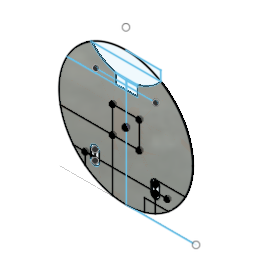
cima (Autodesk Fusion 360 archive; units mm, degrees)
design "BaseChapaCima"
Autodesk Fusion 360 part; units mm, degrees
sketch "Sketch1" plane through (0, 0, 0) normal (0, 0, -1) x (1, 0, 0)
  circle A0 centre (0, 0) radius 240
  line L0 (0.0048, -240) -> (125.0048, -240)
  line L1 (125.0048, -240) -> (125.0048, -204.8751)
  line L2 (1.5986, 239.9947) -> (1.5986, -147.0053)
  line L3 (125.0048, -204.8751) -> (-125.0048, -204.8751)
  arc A1 (125.0048, -204.8751) -> (-125.0048, -204.8751) centre (0, -310.93) ccw
  circle A2 centre (-47.294, 47.294) radius 5
  line L4 (-47.294, 47.294) -> (48.706, 47.294)
  line L5 (48.706, 47.294) -> (48.706, -48.706)
  line L6 (48.706, -48.706) -> (-47.294, -48.706)
  line L7 (-47.294, -48.706) -> (-47.294, 47.294)
  circle A3 centre (48.706, 47.294) radius 5
  circle A4 centre (48.706, -48.706) radius 5
  circle A5 centre (-47.294, -48.706) radius 5
  line L8 (1.5986, 239.9947) -> (251.5986, 239.9947)
  line L9 (-47.294, 47.294) -> (-47.294, 235.294)
  line L10 (-47.294, 47.294) -> (-235.294, 47.294)
  line L11 (105.5391, 215.5493) -> (105.5391, 169.5493)
  line L12 (105.5391, 169.5493) -> (105.5391, 109.5493)
  line L13 (105.5391, 109.5493) -> (213.5391, 109.5493)
  line L14 (105.5391, 109.5493) -> (105.5391, 124.5493)
  line L15 (105.5391, 169.5493) -> (105.5391, 154.5493)
  line L16 (120.5391, 124.5493) -> (120.5391, 154.5493)
  arc A6 (120.5391, 154.5493) -> (90.5391, 154.5493) centre (105.5391, 154.5493) ccw
  line L17 (90.5391, 154.5493) -> (90.5391, 124.5493)
  arc A7 (90.5391, 124.5493) -> (120.5391, 124.5493) centre (105.5391, 124.5493) ccw
  line L18 (105.5391, 124.5493) -> (105.5391, 154.5493) construction
  line L19 (1.5986, -147.0053) -> (41.5986, -147.0053)
  line L20 (41.5986, -147.0053) -> (41.5986, -152.3633)
  line L21 (1.5986, -147.0053) -> (1.5986, -115.0053)
  line L22 (1.5986, -115.0053) -> (-38.4014, -115.0053)
  line L23 (41.5986, -152.3633) -> (-38.4014, -152.3633)
  line L24 (-38.4014, -152.3633) -> (-38.4014, -115.0053)
  line L25 (-38.4014, -115.0053) -> (41.5986, -115.0053)
  line L26 (41.5986, -115.0053) -> (41.5986, -152.3633)
  line L27 (-145.8667, 190.5857) -> (-145.8667, 148.0857)
  line L28 (-145.8667, 148.0857) -> (-188.8667, 148.0857)
  circle A8 centre (-145.8667, 148.0857) radius 5
  line L29 (-145.8667, 148.0857) -> (-110.8667, 148.0857)
  line L30 (-110.8667, 159.0843) -> (-110.8667, 124.0843)
  line L31 (-125.8667, 159.0843) -> (-125.8667, 124.0843)
  arc A9 (-125.8667, 124.0843) -> (-95.8667, 124.0843) centre (-110.8667, 124.0843) ccw
  line L32 (-95.8667, 124.0843) -> (-95.8667, 159.0843)
  arc A10 (-95.8667, 159.0843) -> (-125.8667, 159.0843) centre (-110.8667, 159.0843) ccw
  line L33 (-110.8667, 159.0843) -> (-110.8667, 124.0843) construction
  line L34 (-110.8667, 148.0857) -> (-110.8667, 159.0843)
  line L35 (-107.1508, -115.0053) -> (-107.5583, -130.5)
  circle A11 centre (-107.5583, -130.5) radius 5
  line L36 (-38.4014, -115.0053) -> (-210.6508, -115.0053)
  line L37 (-210.6508, -115.0053) -> (-107.1508, -115.0053)
  line L38 (152.5158, 185.3077) -> (67.5158, 185.3077)
  line L39 (67.5158, 185.3077) -> (67.5158, 230.3077)
  line L40 (-107.5583, -130.5) -> (107.9417, -130.5)
  circle A12 centre (107.9417, -130.5) radius 5
  line L41 (-145.8667, 148.0857) -> (149.1333, 148.0857)
  circle A13 centre (149.1333, 148.0857) radius 5
  dimension "d1" = 480
  dimension "d2" = 125
  dimension "d3" = 387
  dimension "d7" = 10
  dimension "d8" = 96
  dimension "d9" = 96
  dimension "d10" = 10
  dimension "d11" = 10
  dimension "d12" = 10
  dimension "d13" = 250
  dimension "d14" = 188
  dimension "d15" = 188
  dimension "d16" = 46
  dimension "d17" = 60
  dimension "d18" = 108
  dimension "d19" = 15
  dimension "d20" = 15
  dimension "d21" = 30
  dimension "d22" = 40
  dimension "d23" = 32
  dimension "d24" = 40
  dimension "d25" = 42.5
  dimension "d26" = 43
  dimension "d27" = 10
  dimension "d28" = 35
  dimension "d29" = 35
  dimension "d30" = 30
  dimension "d32" = 15.5
  dimension "d33" = 10
  dimension "d34" = 103.5
  dimension "d35" = 85
  dimension "d36" = 45
  dimension "d40" = 215.5
  dimension "d41" = 10
  dimension "d42" = 295
  dimension "d43" = 10
  constraint coincident A0.centre origin
  constraint coincident A0 L0.start
  constraint horizontal L0
  constraint coincident A0 L1.end
  constraint perpendicular L0 L1
  constraint coincident A0 L2.start
  constraint vertical L2
  constraint coincident A0 L3.end
  constraint perpendicular L1 L3
  constraint coincident L2.end A1
  constraint horizontal L4
  constraint vertical L5
  constraint horizontal L6
  constraint vertical L7
  constraint coincident A2.centre L4.start
  constraint coincident L4.end L5.start
  constraint coincident L5.end L6.start
  constraint coincident L6.end L7.start
  constraint perpendicular L2 L8
  constraint coincident A0 L9.end
  constraint parallel L7 L9
  constraint coincident A0 L10.end
  constraint perpendicular L9 L10
  constraint coincident A0 L11.start
  constraint vertical L11
  constraint parallel L11 L12
  constraint perpendicular L12 L13
  constraint coincident A0 L13.end
  constraint perpendicular L13 L14
  constraint parallel L12 L15
  constraint tangent L16 A6
  constraint tangent A6 L17
  constraint parallel L16 L17
  constraint tangent L17 A7
  constraint tangent L16 A7
  constraint coincident L15.end A6.centre
  constraint parallel L15 L18
  constraint coincident L14.end A7.centre
  constraint perpendicular L2 L19
  constraint coincident A1 L20.end
  constraint perpendicular L19 L20
  constraint perpendicular L19 L21
  constraint perpendicular L2 L22
  constraint horizontal L23
  constraint vertical L24
  constraint horizontal L25
  constraint vertical L26
  constraint coincident A0 L27.start
  constraint parallel L2 L27
  constraint coincident A0 L28.end
  constraint perpendicular L27 L28
  constraint coincident L27.end L28.start
  constraint perpendicular L27 L29
  constraint tangent L31 A9
  constraint tangent A9 L32
  constraint parallel L31 L32
  constraint tangent L32 A10
  constraint tangent L31 A10
  constraint coincident L30.end A9.centre
  constraint perpendicular L29 L33
  constraint coincident L30.start A10.centre
  constraint coincident L35.end A11.centre
  constraint coincident A0 L36.end
  constraint perpendicular L24 L36
  constraint parallel L36 L37
  constraint coincident L35.start L37.end
  constraint coincident A0 L38.start
  constraint horizontal L38
  constraint coincident A0 L39.end
  constraint perpendicular L38 L39
  constraint horizontal L40
  constraint coincident L40.end A12.centre
  constraint perpendicular L34 L41
  constraint coincident L41.end A13.centre
  constraint parallel L4 L41
  measures "d1" diameter of A0
  measures "d2" distance of L0.start L0.end
  measures "d3" distance of L2.start L2.end
  measures "d7" diameter of A2
  measures "d8" distance of A2.centre L4.end
  measures "d9" distance of A2.centre L6.end
  measures "d10" diameter of A3
  measures "d11" diameter of A4
  measures "d12" diameter of A5
  measures "d13" distance of L2.start L8.end
  measures "d14" distance of A2.centre L10.end
  measures "d15" distance of A2.centre L9.end
  measures "d16" distance of L11.start L11.end
  measures "d17" distance of L11.end L12.end
  measures "d18" distance of L12.end L13.end
  measures "d19" distance of L12.end L14.end
  measures "d20" distance of L11.end L15.end
  measures "d21" diameter of A6
  measures "d22" distance of L2.end L19.end
  measures "d23" distance of L2.end L21.end
  measures "d24" distance of L21.end L22.end
  measures "d25" distance of L27.start L27.end
  measures "d26" distance of L27.end L28.end
  measures "d27" diameter of A8
  measures "d28" distance of L27.end L29.end
  measures "d29" distance of L30.start L30.end
  measures "d30" diameter of A9
  measures "d32" distance of L35.start L35.end
  measures "d33" diameter of A11
  measures "d34" distance of L36.end L35.start
  measures "d35" distance of L38.start L38.end
  measures "d36" distance of L38.end L39.end
  measures "d40" distance of L35.end L40.end
  measures "d41" diameter of A12
  measures "d42" distance of L27.end L41.end
  measures "d43" diameter of A13
extrude "Extrude3" add sketch "Sketch1" along normal blind 3 contours A0 L2 A1 L4 L5 L6 A3 A4 L13 L17 A7 L20 L25 L26 L41 | A0 L11 L13 L16 A6 A7 L38 | A0 L11 L38 | A0 A1 L24 L35 A11 L36 L37 L40 | A0 L11 L38 L39 | A0 L2 L11 A6 L17 L38 L39 L41 | A0 L2 A2 L6 L7 A5 L10 L22 L25 L36 L37 | A0 A2 L9 L10 L28 A8 L29 L31 A9 L32 L41 | L24 L35 A11 L36 L40 | A0 L2 L9 L41 | L2 A2 L4 L9 L41 | A0 L27 L28 A8 | A0 L9 L27 A8 L29 L31 L32 A10 L41 | L2 L4 L5 L6 A3 A4 | L2 A2 L4 L6 L7 A5
equation "d2 = ( 250 / 2 ) * 1 mm"
equation "d3 = 355 mm + 32 mm"
